Autodesk Fusion 360 part; units mm, degrees
(part 3 of 5)
  spline S141 degree 3 poles (-283.1906, 51.225) (-283.1957, 51.1131) (-283.2051, 50.9053) (-283.324, 50.7357) (-283.3788, 50.6575) knots 0 0 0 0 0.032809 0.060899 0.060899 0.060899 0.060899
  spline S142 degree 3 poles (-283.3788, 50.6575) (-283.4474, 50.5986) (-283.5878, 50.478) (-283.7726, 50.4631) (-283.8672, 50.4556) knots 0 0 0 0 0.026399 0.05408 0.05408 0.05408 0.05408
  spline S143 degree 3 poles (-283.8672, 50.4556) (-283.959, 50.4631) (-284.1388, 50.4779) (-284.2752, 50.5957) (-284.342, 50.6534) knots 0 0 0 0 0.026858 0.052633 0.052633 0.052633 0.052633
  spline S144 degree 3 poles (-284.342, 50.6534) (-284.3956, 50.7301) (-284.512, 50.8965) (-284.5212, 51.1002) (-284.5262, 51.21) knots 0 0 0 0 0.027523 0.05971 0.05971 0.05971 0.05971
  spline S145 degree 3 poles (-284.5262, 51.21) (-284.5261, 51.2191) (-284.5259, 51.2409) (-284.5252, 51.2627) (-284.5248, 51.2755) knots 0 0 0 0 0.002729 0.00655 0.00655 0.00655 0.00655
  line L105 (-284.5248, 51.2755) -> (-283.4443, 51.2755)
  spline S146 degree 3 poles (-283.4443, 51.2755) (-283.4514, 51.3482) (-283.4645, 51.4824) (-283.5433, 51.5913) (-283.5794, 51.6411) knots 0 0 0 0 0.021465 0.039604 0.039604 0.039604 0.039604
  spline S147 degree 3 poles (-283.5794, 51.6411) (-283.6226, 51.6781) (-283.7099, 51.7528) (-283.8244, 51.7629) (-283.8822, 51.768) knots 0 0 0 0 0.016633 0.033577 0.033577 0.033577 0.033577
  line L106 (-285.0691, 51.1786) -> (-285.0691, 51.9371)
  line L107 (-285.0691, 51.9371) -> (-284.8236, 51.9371)
  line L108 (-284.8236, 51.9371) -> (-284.8236, 50.4883)
  line L109 (-284.8236, 50.4883) -> (-285.0446, 50.4883)
  line L110 (-285.0446, 50.4883) -> (-285.0446, 50.7079)
  spline S148 degree 3 poles (-285.0446, 50.7079) (-285.0692, 50.6633) (-285.1111, 50.5874) (-285.1746, 50.5288) (-285.2008, 50.5047) knots 0 0 0 0 0.015158 0.025781 0.025781 0.025781 0.025781
  spline S149 degree 3 poles (-285.2008, 50.5047) (-285.2252, 50.4904) (-285.2739, 50.4618) (-285.3303, 50.4576) (-285.3584, 50.4556) knots 0 0 0 0 0.008374 0.016702 0.016702 0.016702 0.016702
  spline S150 degree 3 poles (-285.3584, 50.4556) (-285.4009, 50.4595) (-285.4906, 50.4677) (-285.5693, 50.5116) (-285.6107, 50.5347) knots 0 0 0 0 0.012672 0.02671 0.02671 0.02671 0.02671
  line L111 (-285.6107, 50.5347) -> (-285.5262, 50.7625)
  spline S151 degree 3 poles (-285.5262, 50.7625) (-285.4968, 50.747) (-285.4403, 50.7172) (-285.3766, 50.7119) (-285.3461, 50.7093) knots 0 0 0 0 0.009849 0.018951 0.018951 0.018951 0.018951
  spline S152 degree 3 poles (-285.3461, 50.7093) (-285.3199, 50.7113) (-285.2677, 50.7154) (-285.2235, 50.7436) (-285.2015, 50.7577) knots 0 0 0 0 0.007735 0.015463 0.015463 0.015463 0.015463
  spline S153 degree 3 poles (-285.2015, 50.7577) (-285.1815, 50.7759) (-285.1403, 50.8133) (-285.1203, 50.8653) (-285.1101, 50.8921) knots 0 0 0 0 0.007973 0.016455 0.016455 0.016455 0.016455
  spline S154 degree 3 poles (-285.1101, 50.8921) (-285.0981, 50.9376) (-285.0735, 51.0315) (-285.0706, 51.1285) (-285.0691, 51.1786) knots 0 0 0 0 0.01405 0.029024 0.029024 0.029024 0.029024
  line L112 (-278.1333, 51.124) -> (-278.1333, 51.9371)
  line L113 (-278.1333, 51.9371) -> (-277.8686, 51.9371)
  line L114 (-277.8686, 51.9371) -> (-277.8686, 49.9371)
  line L115 (-277.8686, 49.9371) -> (-278.623, 49.9371)
  spline S155 degree 3 poles (-278.623, 49.9371) (-278.6817, 49.9373) (-278.7835, 49.9376) (-278.8844, 49.9507) (-278.9272, 49.9562) knots 0 0 0 0 0.017571 0.030509 0.030509 0.030509 0.030509
  spline S156 degree 3 poles (-278.9272, 49.9562) (-278.9734, 49.9656) (-279.0608, 49.9833) (-279.1378, 50.0284) (-279.1742, 50.0497) knots 0 0 0 0 0.014001 0.026564 0.026564 0.026564 0.026564
  spline S157 degree 3 poles (-279.1742, 50.0497) (-279.2061, 50.0756) (-279.2722, 50.1294) (-279.3132, 50.2041) (-279.3345, 50.2427) knots 0 0 0 0 0.012214 0.025303 0.025303 0.025303 0.025303
  spline S158 degree 3 poles (-279.3345, 50.2427) (-279.3522, 50.2856) (-279.3883, 50.373) (-279.3929, 50.4675) (-279.3952, 50.5156) knots 0 0 0 0 0.013801 0.028138 0.028138 0.028138 0.028138
  spline S159 degree 3 poles (-279.3952, 50.5156) (-279.3889, 50.5968) (-279.3765, 50.7566) (-279.2802, 50.8845) (-279.2328, 50.9474) knots 0 0 0 0 0.023898 0.046996 0.046996 0.046996 0.046996
  spline S160 degree 3 poles (-279.2328, 50.9474) (-279.1593, 50.9986) (-278.9848, 51.1201) (-278.7703, 51.1226) (-278.6462, 51.124) knots 0 0 0 0 0.026356 0.062507 0.062507 0.062507 0.062507
  line L116 (-278.6462, 51.124) -> (-278.1333, 51.124)
  spline S161 degree 3 poles (-257.0244, 103.3904) (-257.0362, 103.3956) (-257.0628, 103.4073) (-257.092, 103.4078) (-257.1083, 103.4081) knots 0 0 0 0 0.003804 0.008651 0.008651 0.008651 0.008651
  spline S162 degree 3 poles (-257.1083, 103.4081) (-257.1242, 103.4076) (-257.1603, 103.4063) (-257.196, 103.4014) (-257.2161, 103.3986) knots 0 0 0 0 0.004747 0.010826 0.010826 0.010826 0.010826
  line L117 (-257.2161, 103.3986) -> (-257.2516, 103.6155)
  spline S163 degree 3 poles (-257.2516, 103.6155) (-257.219, 103.6219) (-257.1576, 103.6338) (-257.0952, 103.6362) (-257.0661, 103.6373) knots 0 0 0 0 0.009958 0.018706 0.018706 0.018706 0.018706
  spline S164 degree 3 poles (-257.0661, 103.6373) (-257.0259, 103.6366) (-256.954, 103.6352) (-256.8879, 103.6073) (-256.8587, 103.595) knots 0 0 0 0 0.011916 0.021334 0.021334 0.021334 0.021334
  spline S165 degree 3 poles (-256.8587, 103.595) (-256.8361, 103.5802) (-256.7925, 103.5516) (-256.7672, 103.5059) (-256.755, 103.4839) knots 0 0 0 0 0.007958 0.015408 0.015408 0.015408 0.015408
  spline S166 degree 3 poles (-256.755, 103.4839) (-256.7464, 103.4484) (-256.7233, 103.3534) (-256.7243, 103.2553) (-256.725, 103.194) knots 0 0 0 0 0.010927 0.02924 0.02924 0.02924 0.02924
  line L118 (-256.725, 103.194) -> (-256.725, 102.3604)
  line L119 (-256.725, 102.3604) -> (-256.5449, 102.3604)
  line L120 (-256.5449, 102.3604) -> (-256.5449, 102.1694)
  line L121 (-256.5449, 102.1694) -> (-256.725, 102.1694)
  line L122 (-256.725, 102.1694) -> (-256.725, 101.8106)
  line L123 (-256.725, 101.8106) -> (-256.9692, 101.6633)
  line L124 (-256.9692, 101.6633) -> (-256.9692, 102.1694)
  line L125 (-256.9692, 102.1694) -> (-257.2161, 102.1694)
  line L126 (-257.2161, 102.1694) -> (-257.2161, 102.3604)
  line L127 (-257.2161, 102.3604) -> (-256.9692, 102.3604)
  line L128 (-256.9692, 102.3604) -> (-256.9692, 103.2076)
  spline S167 degree 3 poles (-256.9692, 103.2076) (-256.9688, 103.2365) (-256.9683, 103.2821) (-256.9784, 103.3265) (-256.9822, 103.3427) knots 0 0 0 0 0.008635 0.013608 0.013608 0.013608 0.013608
  spline S168 degree 3 poles (-256.9822, 103.3427) (-256.9872, 103.3522) (-256.9975, 103.3715) (-257.0154, 103.384) (-257.0244, 103.3904) knots 0 0 0 0 0.003189 0.00646 0.00646 0.00646 0.00646
  spline S169 degree 3 poles (-252.8144, 103.5848) (-252.7657, 103.5945) (-252.6592, 103.6158) (-252.5506, 103.6174) (-252.4917, 103.6182) knots 0 0 0 0 0.014862 0.032497 0.032497 0.032497 0.032497
  line L129 (-252.4917, 103.6182) -> (-251.7291, 103.6182)
  line L130 (-251.7291, 103.6182) -> (-251.7291, 101.6182)
  line L131 (-251.7291, 101.6182) -> (-252.4794, 101.6182)
  spline S170 degree 3 poles (-252.4794, 101.6182) (-252.5489, 101.6195) (-252.6746, 101.6218) (-252.7938, 101.6613) (-252.8471, 101.6789) knots 0 0 0 0 0.020707 0.037453 0.037453 0.037453 0.037453
  spline S171 degree 3 poles (-252.8471, 101.6789) (-252.8907, 101.7018) (-252.9775, 101.7473) (-253.0353, 101.8265) (-253.064, 101.8658) knots 0 0 0 0 0.014555 0.028975 0.028975 0.028975 0.028975
  spline S172 degree 3 poles (-253.064, 101.8658) (-253.0869, 101.9079) (-253.1317, 101.9904) (-253.1389, 102.084) (-253.1425, 102.1298) knots 0 0 0 0 0.014187 0.027818 0.027818 0.027818 0.027818
  spline S173 degree 3 poles (-253.1425, 102.1298) (-253.1394, 102.1721) (-253.1334, 102.2575) (-253.0932, 102.3331) (-253.0729, 102.3713) knots 0 0 0 0 0.01257 0.025379 0.025379 0.025379 0.025379
  spline S174 degree 3 poles (-253.0729, 102.3713) (-253.0458, 102.4077) (-252.9891, 102.4838) (-252.9061, 102.53) (-252.8628, 102.5541) knots 0 0 0 0 0.013451 0.028132 0.028132 0.028132 0.028132
  spline S175 degree 3 poles (-252.8628, 102.5541) (-252.919, 102.574) (-253.0268, 102.6121) (-253.1046, 102.6956) (-253.1418, 102.7356) knots 0 0 0 0 0.017587 0.033722 0.033722 0.033722 0.033722
  spline S176 degree 3 poles (-253.1418, 102.7356) (-253.1702, 102.7808) (-253.2284, 102.8734) (-253.2356, 102.9826) (-253.2393, 103.0384) knots 0 0 0 0 0.015782 0.032266 0.032266 0.032266 0.032266
  spline S177 degree 3 poles (-253.2393, 103.0384) (-253.237, 103.0842) (-253.2323, 103.1747) (-253.1973, 103.2584) (-253.18, 103.2997) knots 0 0 0 0 0.013638 0.026971 0.026971 0.026971 0.026971
  spline S178 degree 3 poles (-253.18, 103.2997) (-253.1599, 103.3369) (-253.1218, 103.4076) (-253.0617, 103.4608) (-253.0333, 103.4859) knots 0 0 0 0 0.012583 0.02387 0.02387 0.02387 0.02387
  spline S179 degree 3 poles (-253.0333, 103.4859) (-253.0013, 103.5067) (-252.9333, 103.5507) (-252.8555, 103.573) (-252.8144, 103.5848) knots 0 0 0 0 0.011395 0.024144 0.024144 0.024144 0.024144
  spline S180 degree 3 poles (-269.284, 103.5337) (-269.2388, 103.4878) (-269.1427, 103.3903) (-269.1115, 103.2566) (-269.095, 103.1858) knots 0 0 0 0 0.01895 0.040278 0.040278 0.040278 0.040278
  line L132 (-269.095, 103.1858) -> (-269.3379, 103.1476)
  spline S181 degree 3 poles (-269.713, 103.4491) (-269.7635, 103.4479) (-269.8534, 103.4458) (-269.9303, 103.4002) (-269.9641, 103.3802) knots 0 0 0 0 0.014834 0.026419 0.026419 0.026419 0.026419
  spline S182 degree 3 poles (-269.9641, 103.3802) (-269.9879, 103.3569) (-270.0338, 103.3122) (-270.042, 103.2489) (-270.0459, 103.2185) knots 0 0 0 0 0.009682 0.0186 0.0186 0.0186 0.0186
  spline S183 degree 3 poles (-269.4572, 102.166) (-269.4912, 102.1574) (-269.5609, 102.1399) (-269.6326, 102.1378) (-269.6694, 102.1367) knots 0 0 0 0 0.010482 0.021472 0.021472 0.021472 0.021472
  spline S184 degree 3 poles (-269.6694, 102.1367) (-269.7232, 102.1382) (-269.8253, 102.1412) (-269.9227, 102.1715) (-269.9688, 102.1858) knots 0 0 0 0 0.01606 0.030471 0.030471 0.030471 0.030471
  spline S185 degree 3 poles (-268.4797, 103.3781) (-268.5106, 103.349) (-268.5781, 103.2853) (-268.6125, 103.1987) (-268.6312, 103.1517) knots 0 0 0 0 0.012573 0.027537 0.027537 0.027537 0.027537
  line L133 (-268.6312, 103.1517) -> (-268.8849, 103.183)
  line L134 (-252.4198, 62.5518) -> (-336.4198, 62.5518)
  line L135 (-336.4198, 62.5518) -> (-336.4198, 86.5518)
  line L136 (-336.4198, 86.5518) -> (-252.4198, 86.5518)
  line L137 (-252.4198, 86.5518) -> (-252.4198, 62.5518)
  line L138 (-334.4198, 84.5518) -> (-254.4198, 84.5518)
  line L139 (-254.4198, 84.5518) -> (-254.4198, 64.5518)
  line L140 (-254.4198, 64.5518) -> (-334.4198, 64.5518)
  line L141 (-334.4198, 64.5518) -> (-334.4198, 84.5518)
  line L142 (-254.4198, 64.5518) -> (-264.4198, 64.5518)
  line L143 (-264.4198, 64.5518) -> (-264.4198, 74.5518)
  line L144 (-264.4198, 74.5518) -> (-254.4198, 74.5518)
  line L145 (-254.4198, 74.5518) -> (-254.4198, 64.5518)
  line L146 (-264.4198, 74.5518) -> (-274.4198, 74.5518)
  line L147 (-274.4198, 74.5518) -> (-274.4198, 64.5518)
  line L148 (-274.4198, 64.5518) -> (-264.4198, 64.5518)
  line L149 (-264.4198, 64.5518) -> (-264.4198, 74.5518)
  line L150 (-274.4198, 74.5518) -> (-284.4198, 74.5518)
  line L151 (-284.4198, 74.5518) -> (-284.4198, 64.5518)
  line L152 (-284.4198, 64.5518) -> (-274.4198, 64.5518)
  line L153 (-274.4198, 64.5518) -> (-274.4198, 74.5518)
  line L154 (-284.4198, 74.5518) -> (-294.4198, 74.5518)
  line L155 (-294.4198, 74.5518) -> (-294.4198, 64.5518)
  line L156 (-294.4198, 64.5518) -> (-284.4198, 64.5518)
  line L157 (-284.4198, 64.5518) -> (-284.4198, 74.5518)
  line L158 (-294.4198, 74.5518) -> (-304.4198, 74.5518)
  line L159 (-304.4198, 74.5518) -> (-304.4198, 64.5518)
  line L160 (-304.4198, 64.5518) -> (-294.4198, 64.5518)
  line L161 (-294.4198, 64.5518) -> (-294.4198, 74.5518)
  line L162 (-304.4198, 74.5518) -> (-314.4198, 74.5518)
  line L163 (-314.4198, 74.5518) -> (-314.4198, 64.5518)
  line L164 (-314.4198, 64.5518) -> (-304.4198, 64.5518)
  line L165 (-304.4198, 64.5518) -> (-304.4198, 74.5518)
  line L166 (-314.4198, 74.5518) -> (-324.4198, 74.5518)
  line L167 (-324.4198, 64.5518) -> (-314.4198, 64.5518)
  line L168 (-314.4198, 64.5518) -> (-314.4198, 74.5518)
  line L169 (-324.4198, 74.5518) -> (-334.4198, 74.5518)
  line L170 (-334.4198, 74.5518) -> (-334.4198, 64.5518)
  line L171 (-334.4198, 64.5518) -> (-324.4198, 64.5518)
  line L172 (-254.4198, 64.5518) -> (-264.4198, 64.5518)
  line L173 (-264.4198, 64.5518) -> (-264.4198, 74.5518)
  line L174 (-264.4198, 74.5518) -> (-254.4198, 74.5518)
  line L175 (-254.4198, 74.5518) -> (-254.4198, 64.5518)
  line L176 (-254.4198, 64.5518) -> (-264.4198, 74.5518)
  line L177 (-264.4198, 74.5518) -> (-274.4198, 64.5518)
  line L178 (-274.4198, 64.5518) -> (-284.4198, 74.5518)
  line L179 (-284.4198, 74.5518) -> (-294.4198, 64.5518)
  line L180 (-294.4198, 64.5518) -> (-304.4198, 74.5518)
  line L181 (-304.4198, 74.5518) -> (-314.4198, 64.5518)
  line L182 (-314.4198, 64.5518) -> (-324.4198, 74.5518)
  line L183 (-324.4198, 74.5518) -> (-334.4198, 64.5518)
  line L184 (-262.0056, 73.5518) -> (-255.4198, 73.5518)
  line L185 (-255.4198, 73.5518) -> (-255.4198, 66.966)
  line L186 (-255.4198, 66.966) -> (-262.0056, 73.5518)
  line L187 (-256.834, 65.5518) -> (-263.4198, 72.1376)
  line L188 (-263.4198, 65.5518) -> (-263.4198, 72.1376)
  line L189 (-256.834, 65.5518) -> (-263.4198, 65.5518)
  line L190 (-272.0056, 65.5518) -> (-265.4198, 65.5518)
  line L191 (-265.4198, 65.5518) -> (-265.4198, 72.1376)
  line L192 (-265.4198, 72.1376) -> (-272.0056, 65.5518)
  line L193 (-273.4198, 73.5518) -> (-273.4198, 66.966)
  line L194 (-266.834, 73.5518) -> (-273.4198, 66.966)
  line L195 (-266.834, 73.5518) -> (-273.4198, 73.5518)
  line L196 (-275.4198, 73.5518) -> (-275.4198, 66.966)
  line L197 (-275.4198, 66.966) -> (-282.0056, 73.5518)
  line L198 (-275.4198, 73.5518) -> (-282.0056, 73.5518)
  line L199 (-283.4198, 72.1376) -> (-283.4198, 65.5518)
  line L200 (-283.4198, 65.5518) -> (-276.834, 65.5518)
  line L201 (-276.834, 65.5518) -> (-283.4198, 72.1376)
  line L202 (-292.0056, 65.5518) -> (-285.4198, 65.5518)
  line L203 (-285.4198, 65.5518) -> (-285.4198, 72.1376)
  line L204 (-285.4198, 72.1376) -> (-292.0056, 65.5518)
  line L205 (-293.4198, 73.5518) -> (-293.4198, 66.966)
  line L206 (-286.834, 73.5518) -> (-293.4198, 66.966)
  line L207 (-286.834, 73.5518) -> (-293.4198, 73.5518)
  line L208 (-295.4198, 73.5518) -> (-295.4198, 66.966)
  line L209 (-295.4198, 66.966) -> (-302.0056, 73.5518)
  line L210 (-295.4198, 73.5518) -> (-302.0056, 73.5518)
  line L211 (-303.4198, 65.5518) -> (-303.4198, 72.1376)
  line L212 (-304.4198, 64.5518) -> (-304.4198, 65.5518)
  line L213 (-303.4198, 65.5518) -> (-296.834, 65.5518)
  line L214 (-296.834, 65.5518) -> (-303.4198, 72.1376)
  line L215 (-305.4198, 65.5518) -> (-305.4198, 72.1376)
  line L216 (-305.4198, 72.1376) -> (-312.0056, 65.5518)
  line L217 (-312.0056, 65.5518) -> (-305.4198, 65.5518)
  line L218 (-306.834, 73.5518) -> (-313.4198, 73.5518)
  line L219 (-313.4198, 66.966) -> (-313.4198, 73.5518)
  line L220 (-306.834, 73.5518) -> (-313.4198, 66.966)
  line L221 (-315.4198, 73.5518) -> (-322.0056, 73.5518)
  line L222 (-315.4198, 66.966) -> (-322.0056, 73.5518)
  line L223 (-315.4198, 73.5518) -> (-315.4198, 66.966)
  line L224 (-316.834, 65.5518) -> (-323.4198, 72.1376)
  line L225 (-323.4198, 72.1376) -> (-323.4198, 65.5518)
  line L226 (-323.4198, 65.5518) -> (-316.834, 65.5518)
  line L227 (-325.4198, 72.1376) -> (-332.0056, 65.5518)
  line L228 (-325.4198, 72.1376) -> (-325.4198, 65.5518)
  line L229 (-325.4198, 65.5518) -> (-332.0056, 65.5518)
  line L230 (-333.4198, 73.5518) -> (-333.4198, 66.966)
  line L231 (-326.834, 73.5518) -> (-333.4198, 66.966)
  line L232 (-326.834, 73.5518) -> (-333.4198, 73.5518)
  line L233 (-326.834, 75.5518) -> (-333.4198, 75.5518)
  line L234 (-306.834, 75.5518) -> (-313.4198, 75.5518)
  line L235 (-315.4198, 75.5518) -> (-322.0056, 75.5518)
  line L236 (-295.4198, 75.5518) -> (-302.0056, 75.5518)
  line L237 (-286.834, 75.5518) -> (-293.4198, 75.5518)
  line L238 (-275.4198, 75.5518) -> (-282.0056, 75.5518)
  line L239 (-283.4198, 83.5518) -> (-276.834, 83.5518)
  line L240 (-325.4198, 83.5518) -> (-332.0056, 83.5518)
  line L241 (-292.0056, 83.5518) -> (-285.4198, 83.5518)
  line L242 (-303.4198, 83.5518) -> (-296.834, 83.5518)
  line L243 (-256.834, 83.5518) -> (-263.4198, 83.5518)
  line L244 (-325.4198, 76.966) -> (-332.0056, 83.5518)
  line L245 (-323.4198, 83.5518) -> (-316.834, 83.5518)
  line L246 (-266.834, 75.5518) -> (-273.4198, 75.5518)
  line L247 (-333.4198, 75.5518) -> (-333.4198, 82.1376)
  line L248 (-312.0056, 83.5518) -> (-305.4198, 83.5518)
  line L249 (-326.834, 75.5518) -> (-333.4198, 82.1376)
  line L250 (-305.4198, 76.966) -> (-312.0056, 83.5518)
  line L251 (-272.0056, 83.5518) -> (-265.4198, 83.5518)
  line L252 (-276.834, 83.5518) -> (-283.4198, 76.966)
  line L253 (-315.4198, 75.5518) -> (-315.4198, 82.1376)
  line L254 (-255.4198, 82.1376) -> (-262.0056, 75.5518)
  line L255 (-293.4198, 75.5518) -> (-293.4198, 82.1376)
  line L256 (-283.4198, 76.966) -> (-283.4198, 83.5518)
  line L257 (-285.4198, 76.966) -> (-292.0056, 83.5518)
  line L258 (-275.4198, 82.1376) -> (-282.0056, 75.5518)
  line L259 (-275.4198, 75.5518) -> (-275.4198, 82.1376)
  line L260 (-296.834, 83.5518) -> (-303.4198, 76.966)
  line L261 (-323.4198, 76.966) -> (-323.4198, 83.5518)
  line L262 (-285.4198, 83.5518) -> (-285.4198, 76.966)
  line L263 (-273.4198, 75.5518) -> (-273.4198, 82.1376)
  line L264 (-313.4198, 82.1376) -> (-313.4198, 75.5518)
  line L265 (-262.0056, 75.5518) -> (-255.4198, 75.5518)
  line L266 (-286.834, 75.5518) -> (-293.4198, 82.1376)
  line L267 (-255.4198, 75.5518) -> (-255.4198, 82.1376)
  line L268 (-305.4198, 83.5518) -> (-305.4198, 76.966)
  line L269 (-265.4198, 83.5518) -> (-265.4198, 76.966)
  line L270 (-265.4198, 76.966) -> (-272.0056, 83.5518)
  line L271 (-325.4198, 76.966) -> (-325.4198, 83.5518)
  line L272 (-316.834, 83.5518) -> (-323.4198, 76.966)
  line L273 (-266.834, 75.5518) -> (-273.4198, 82.1376)
  line L274 (-256.834, 83.5518) -> (-263.4198, 76.966)
  line L275 (-306.834, 75.5518) -> (-313.4198, 82.1376)
  line L276 (-295.4198, 75.5518) -> (-295.4198, 82.1376)
  line L277 (-303.4198, 83.5518) -> (-303.4198, 76.966)
  line L278 (-263.4198, 83.5518) -> (-263.4198, 76.966)
  line L279 (-295.4198, 82.1376) -> (-302.0056, 75.5518)
  line L280 (-315.4198, 82.1376) -> (-322.0056, 75.5518)
  line L281 (-265.6571, 101.6182) -> (-266.5439, 101.6182)
  spline S186 degree 3 poles (-267.5384, 51.7255) (-267.4544, 51.7234) (-267.2987, 51.7194) (-267.1513, 51.6694) (-267.0834, 51.6464) knots 0 0 0 0 0.025027 0.046416 0.046416 0.046416 0.046416
  spline S187 degree 3 poles (-269.7144, 103.651) (-269.6293, 103.6486) (-269.4757, 103.6442) (-269.3431, 103.5678) (-269.284, 103.5337) knots 0 0 0 0 0.025053 0.045234 0.045234 0.045234 0.045234
  spline S188 degree 3 poles (-269.3379, 103.1476) (-269.3468, 103.1926) (-269.3638, 103.2781) (-269.4235, 103.3414) (-269.4518, 103.3713) knots 0 0 0 0 0.013461 0.025563 0.025563 0.025563 0.025563
  spline S189 degree 3 poles (-269.4518, 103.3713) (-269.4881, 103.3939) (-269.5678, 103.4435) (-269.6619, 103.4471) (-269.713, 103.4491) knots 0 0 0 0 0.012631 0.027679 0.027679 0.027679 0.027679
  spline S190 degree 3 poles (-270.0459, 103.2185) (-270.0428, 103.1922) (-270.0364, 103.1388) (-269.9947, 103.1048) (-269.9736, 103.0875) knots 0 0 0 0 0.007652 0.015492 0.015492 0.015492 0.015492
  spline S191 degree 3 poles (-269.9736, 103.0875) (-269.9445, 103.0745) (-269.8638, 103.0382) (-269.7777, 103.0175) (-269.7226, 103.0043) knots 0 0 0 0 0.009553 0.026493 0.026493 0.026493 0.026493
  spline S192 degree 3 poles (-269.7226, 103.0043) (-269.6457, 102.9851) (-269.5185, 102.9532) (-269.3964, 102.9053) (-269.3481, 102.8863) knots 0 0 0 0 0.023736 0.039299 0.039299 0.039299 0.039299
  spline S193 degree 3 poles (-269.3481, 102.8863) (-269.3157, 102.8686) (-269.2528, 102.8342) (-269.2104, 102.7765) (-269.1898, 102.7485) knots 0 0 0 0 0.010927 0.021211 0.021211 0.021211 0.021211
  spline S194 degree 3 poles (-269.1898, 102.7485) (-269.1741, 102.7183) (-269.1424, 102.6573) (-269.1381, 102.5887) (-269.1359, 102.5541) knots 0 0 0 0 0.010103 0.020373 0.020373 0.020373 0.020373
  spline S195 degree 3 poles (-269.1359, 102.5541) (-269.1377, 102.5225) (-269.1413, 102.46) (-269.1674, 102.403) (-269.1803, 102.3747) knots 0 0 0 0 0.009394 0.018625 0.018625 0.018625 0.018625
  spline S196 degree 3 poles (-269.1803, 102.3747) (-269.1964, 102.3484) (-269.2287, 102.2956) (-269.2769, 102.257) (-269.301, 102.2376) knots 0 0 0 0 0.009191 0.018392 0.018392 0.018392 0.018392
  spline S197 degree 3 poles (-269.301, 102.2376) (-269.3232, 102.2237) (-269.372, 102.1929) (-269.4271, 102.1755) (-269.4572, 102.166) knots 0 0 0 0 0.007816 0.017247 0.017247 0.017247 0.017247
  spline S198 degree 3 poles (-269.9688, 102.1858) (-270.0081, 102.2024) (-270.0811, 102.2333) (-270.1345, 102.2918) (-270.1591, 102.3188) knots 0 0 0 0 0.012608 0.023462 0.023462 0.023462 0.023462
  spline S199 degree 3 poles (-270.1591, 102.3188) (-270.1783, 102.3508) (-270.2199, 102.4204) (-270.2354, 102.5001) (-270.2437, 102.5432) knots 0 0 0 0 0.011092 0.024145 0.024145 0.024145 0.024145
  line L282 (-270.2437, 102.5432) -> (-270.0036, 102.5759)
  spline S200 degree 3 poles (-270.0036, 102.5759) (-269.996, 102.5411) (-269.9813, 102.4735) (-269.9324, 102.4249) (-269.9088, 102.4013) knots 0 0 0 0 0.010457 0.02025 0.02025 0.02025 0.02025
  spline S201 degree 3 poles (-269.9088, 102.4013) (-269.878, 102.3831) (-269.81, 102.3427) (-269.7306, 102.34) (-269.6871, 102.3386) knots 0 0 0 0 0.01057 0.023371 0.023371 0.023371 0.023371
  spline S202 degree 3 poles (-269.6871, 102.3386) (-269.6377, 102.339) (-269.5526, 102.3396) (-269.4772, 102.3783) (-269.4456, 102.3945) knots 0 0 0 0 0.014562 0.025087 0.025087 0.025087 0.025087
  spline S203 degree 3 poles (-269.4456, 102.3945) (-269.4246, 102.4131) (-269.3847, 102.4484) (-269.377, 102.5008) (-269.3733, 102.5255) knots 0 0 0 0 0.00814 0.015395 0.015395 0.015395 0.015395
  spline S204 degree 3 poles (-269.3733, 102.5255) (-269.3746, 102.541) (-269.3772, 102.5723) (-269.3946, 102.5983) (-269.4033, 102.6114) knots 0 0 0 0 0.004598 0.009239 0.009239 0.009239 0.009239
  spline S205 degree 3 poles (-269.4033, 102.6114) (-269.4156, 102.6243) (-269.4423, 102.6526) (-269.4781, 102.6684) (-269.4975, 102.6769) knots 0 0 0 0 0.005284 0.01157 0.01157 0.01157 0.01157
  spline S206 degree 3 poles (-269.4975, 102.6769) (-269.5217, 102.6845) (-269.5935, 102.7071) (-269.6662, 102.7267) (-269.7144, 102.7397) knots 0 0 0 0 0.007605 0.022583 0.022583 0.022583 0.022583
  spline S207 degree 3 poles (-269.7144, 102.7397) (-269.7886, 102.7594) (-269.9115, 102.792) (-270.0307, 102.8361) (-270.078, 102.8536) knots 0 0 0 0 0.023005 0.038118 0.038118 0.038118 0.038118
  spline S208 degree 3 poles (-270.078, 102.8536) (-270.1102, 102.8697) (-270.1733, 102.9012) (-270.2179, 102.9558) (-270.2396, 102.9825) knots 0 0 0 0 0.010681 0.020888 0.020888 0.020888 0.020888
  spline S209 degree 3 poles (-270.2396, 102.9825) (-270.2567, 103.0134) (-270.2928, 103.0787) (-270.2964, 103.1533) (-270.2983, 103.1926) knots 0 0 0 0 0.010453 0.022074 0.022074 0.022074 0.022074
  spline S210 degree 3 poles (-270.2983, 103.1926) (-270.2951, 103.2332) (-270.2887, 103.3156) (-270.2476, 103.3874) (-270.2267, 103.4238) knots 0 0 0 0 0.012054 0.024479 0.024479 0.024479 0.024479
  spline S211 degree 3 poles (-270.2267, 103.4238) (-270.1994, 103.4582) (-270.1431, 103.5295) (-270.0619, 103.5704) (-270.02, 103.5916) knots 0 0 0 0 0.013001 0.026908 0.026908 0.026908 0.026908
  spline S212 degree 3 poles (-270.02, 103.5916) (-269.9725, 103.6089) (-269.8738, 103.6449) (-269.7688, 103.6489) (-269.7144, 103.651) knots 0 0 0 0 0.015065 0.0313 0.0313 0.0313 0.0313
  spline S213 degree 3 poles (-268.2492, 103.4491) (-268.292, 103.4465) (-268.3747, 103.4416) (-268.4455, 103.3988) (-268.4797, 103.3781) knots 0 0 0 0 0.012642 0.024448 0.024448 0.024448 0.024448
  spline S214 degree 3 poles (-268.8849, 103.183) (-268.8616, 103.2523) (-268.8165, 103.3862) (-268.7127, 103.4819) (-268.6626, 103.5282) knots 0 0 0 0 0.021523 0.041652 0.041652 0.041652 0.041652
  spline S215 degree 3 poles (-268.8931, 102.8911) (-268.893, 102.9002) (-268.8928, 102.922) (-268.8921, 102.9438) (-268.8917, 102.9566) knots 0 0 0 0 0.002729 0.00655 0.00655 0.00655 0.00655
  line L283 (-268.8917, 102.9566) -> (-267.8113, 102.9566)
  spline S216 degree 3 poles (-267.8113, 102.9566) (-267.8184, 103.0293) (-267.8314, 103.1635) (-267.9102, 103.2724) (-267.9463, 103.3222) knots 0 0 0 0 0.021465 0.039604 0.039604 0.039604 0.039604
  spline S217 degree 3 poles (-267.9463, 103.3222) (-267.9896, 103.3592) (-268.0769, 103.4339) (-268.1914, 103.444) (-268.2492, 103.4491) knots 0 0 0 0 0.016633 0.033577 0.033577 0.033577 0.033577
  spline S218 degree 3 poles (-266.8222, 103.2021) (-266.7876, 103.1487) (-266.7268, 103.0548) (-266.66, 102.9652) (-266.6312, 102.9266) knots 0 0 0 0 0.019089 0.033538 0.033538 0.033538 0.033538
  spline S219 degree 3 poles (-266.6312, 102.9266) (-266.6086, 102.8983) (-266.5688, 102.8486) (-266.5185, 102.8097) (-266.4968, 102.7929) knots 0 0 0 0 0.010792 0.019015 0.019015 0.019015 0.019015
  spline S220 degree 3 poles (-266.4968, 102.7929) (-266.4772, 102.7812) (-266.4392, 102.7584) (-266.3967, 102.7458) (-266.3761, 102.7397) knots 0 0 0 0 0.006806 0.01324 0.01324 0.01324 0.01324
  spline S221 degree 3 poles (-266.3761, 102.7397) (-266.3563, 102.7369) (-266.3075, 102.7301) (-266.2581, 102.7301) (-266.2287, 102.7301) knots 0 0 0 0 0.005978 0.01478 0.01478 0.01478 0.01478
  line L284 (-272.1892, 103.194) -> (-272.1892, 102.3604)
  line L285 (-272.1892, 102.3604) -> (-272.0091, 102.3604)
  line L286 (-272.0091, 102.3604) -> (-272.0091, 102.1694)
  line L287 (-272.0091, 102.1694) -> (-272.1892, 102.1694)
  line L288 (-272.1892, 102.1694) -> (-272.1892, 101.8106)
  line L289 (-272.1892, 101.8106) -> (-272.4334, 101.6633)
  line L290 (-272.4334, 101.6633) -> (-272.4334, 102.1694)
  line L291 (-272.4334, 102.1694) -> (-272.6803, 102.1694)
  line L292 (-272.6803, 102.1694) -> (-272.6803, 102.3604)
  line L293 (-272.6803, 102.3604) -> (-272.4334, 102.3604)
  line L294 (-272.4334, 102.3604) -> (-272.4334, 103.2076)
  spline S222 degree 3 poles (-272.4463, 103.3427) (-272.4514, 103.3522) (-272.4616, 103.3715) (-272.4795, 103.384) (-272.4886, 103.3904) knots 0 0 0 0 0.003189 0.00646 0.00646 0.00646 0.00646
  spline S223 degree 3 poles (-271.1851, 102.1367) (-271.2768, 102.1442) (-271.4567, 102.159) (-271.593, 102.2768) (-271.6598, 102.3345) knots 0 0 0 0 0.026858 0.052633 0.052633 0.052633 0.052633
  spline S224 degree 3 poles (-271.6598, 102.3345) (-271.7135, 102.4112) (-271.8298, 102.5776) (-271.839, 102.7813) (-271.844, 102.8911) knots 0 0 0 0 0.027523 0.05971 0.05971 0.05971 0.05971
  spline S225 degree 3 poles (-271.844, 102.8911) (-271.8439, 102.9002) (-271.8437, 102.922) (-271.843, 102.9438) (-271.8426, 102.9566) knots 0 0 0 0 0.002729 0.00655 0.00655 0.00655 0.00655
  line L295 (-271.8426, 102.9566) -> (-270.7621, 102.9566)
  spline S226 degree 3 poles (-267.0834, 51.6464) (-267.0258, 51.6171) (-266.912, 51.5591) (-266.834, 51.4582) (-266.7955, 51.4083) knots 0 0 0 0 0.019136 0.037772 0.037772 0.037772 0.037772
  spline S227 degree 3 poles (-272.6639, 51.4786) (-272.6028, 51.5502) (-272.4816, 51.6924) (-272.2962, 51.7136) (-272.2041, 51.7242) knots 0 0 0 0 0.027153 0.053891 0.053891 0.053891 0.053891
  spline S228 degree 3 poles (-272.2041, 51.7242) (-272.1624, 51.7222) (-272.08, 51.7184) (-272.0028, 51.6894) (-271.9647, 51.6751) knots 0 0 0 0 0.012458 0.024577 0.024577 0.024577 0.024577
  spline S229 degree 3 poles (-271.9647, 51.6751) (-271.9308, 51.6587) (-271.8677, 51.6281) (-271.8212, 51.5758) (-271.7996, 51.5516) knots 0 0 0 0 0.01116 0.020794 0.020794 0.020794 0.020794
  spline S230 degree 3 poles (-271.7996, 51.5516) (-271.7829, 51.5246) (-271.7477, 51.4681) (-271.7321, 51.4034) (-271.7239, 51.3695) knots 0 0 0 0 0.009458 0.019838 0.019838 0.019838 0.019838
  spline S231 degree 3 poles (-271.7239, 51.3695) (-271.7196, 51.3384) (-271.709, 51.2624) (-271.7089, 51.1856) (-271.7089, 51.1403) knots 0 0 0 0 0.009413 0.022992 0.022992 0.022992 0.022992
  line L296 (-271.7089, 51.1403) -> (-271.7089, 50.2426)
  line L297 (-271.7089, 50.2426) -> (-271.9545, 50.2426)
  line L298 (-271.9545, 50.2426) -> (-271.9545, 51.0461)
  spline S232 degree 3 poles (-271.9545, 51.0461) (-271.9542, 51.0999) (-271.9538, 51.1867) (-271.9652, 51.2726) (-271.9695, 51.3053) knots 0 0 0 0 0.016103 0.02599 0.02599 0.02599 0.02599
  spline S233 degree 3 poles (-271.9695, 51.3053) (-271.9791, 51.3357) (-271.9981, 51.3954) (-272.0448, 51.437) (-272.0677, 51.4575) knots 0 0 0 0 0.009371 0.018407 0.018407 0.018407 0.018407
  spline S234 degree 3 poles (-272.0677, 51.4575) (-272.095, 51.4736) (-272.1521, 51.5073) (-272.2185, 51.5109) (-272.2533, 51.5127) knots 0 0 0 0 0.009358 0.019615 0.019615 0.019615 0.019615
  spline S235 degree 3 poles (-272.2533, 51.5127) (-272.2896, 51.5103) (-272.3625, 51.5055) (-272.4278, 51.4726) (-272.4606, 51.4561) knots 0 0 0 0 0.010803 0.021692 0.021692 0.021692 0.021692
  spline S236 degree 3 poles (-273.4129, 51.2208) (-273.4218, 51.2658) (-273.4388, 51.3513) (-273.4985, 51.4146) (-273.5268, 51.4445) knots 0 0 0 0 0.013461 0.025563 0.025563 0.025563 0.025563
  spline S237 degree 3 poles (-273.5268, 51.4445) (-273.5631, 51.4671) (-273.6428, 51.5167) (-273.7369, 51.5203) (-273.788, 51.5223) knots 0 0 0 0 0.012631 0.027679 0.027679 0.027679 0.027679
  spline S238 degree 3 poles (-273.788, 51.5223) (-273.8385, 51.5211) (-273.9284, 51.519) (-274.0053, 51.4734) (-274.0391, 51.4534) knots 0 0 0 0 0.014834 0.026419 0.026419 0.026419 0.026419
  spline S239 degree 3 poles (-274.0391, 51.4534) (-274.0629, 51.4301) (-274.1088, 51.3854) (-274.117, 51.3221) (-274.1209, 51.2917) knots 0 0 0 0 0.009682 0.0186 0.0186 0.0186 0.0186
  spline S240 degree 3 poles (-274.1209, 51.2917) (-274.1178, 51.2653) (-274.1114, 51.212) (-274.0697, 51.1779) (-274.0486, 51.1607) knots 0 0 0 0 0.007652 0.015492 0.015492 0.015492 0.015492
  spline S241 degree 3 poles (-274.0486, 51.1607) (-274.0195, 51.1477) (-273.9388, 51.1114) (-273.8527, 51.0907) (-273.7976, 51.0775) knots 0 0 0 0 0.009553 0.026493 0.026493 0.026493 0.026493
  spline S242 degree 3 poles (-273.7976, 51.0775) (-273.7207, 51.0583) (-273.5935, 51.0264) (-273.4714, 50.9785) (-273.4231, 50.9595) knots 0 0 0 0 0.023737 0.039299 0.039299 0.039299 0.039299
  spline S243 degree 3 poles (-273.4231, 50.9595) (-273.3907, 50.9418) (-273.3278, 50.9074) (-273.2854, 50.8497) (-273.2648, 50.8217) knots 0 0 0 0 0.010927 0.021211 0.021211 0.021211 0.021211
  spline S244 degree 3 poles (-273.2648, 50.8217) (-273.2491, 50.7915) (-273.2174, 50.7305) (-273.2131, 50.6619) (-273.211, 50.6273) knots 0 0 0 0 0.010103 0.020373 0.020373 0.020373 0.020373
  spline S245 degree 3 poles (-273.211, 50.6273) (-273.2127, 50.5957) (-273.2163, 50.5331) (-273.2424, 50.4762) (-273.2553, 50.4479) knots 0 0 0 0 0.009394 0.018625 0.018625 0.018625 0.018625
  spline S246 degree 3 poles (-273.2553, 50.4479) (-273.2714, 50.4216) (-273.3037, 50.3688) (-273.3519, 50.3301) (-273.376, 50.3108) knots 0 0 0 0 0.009191 0.018392 0.018392 0.018392 0.018392
  spline S247 degree 3 poles (-273.376, 50.3108) (-273.3982, 50.2969) (-273.447, 50.2661) (-273.5021, 50.2487) (-273.5322, 50.2392) knots 0 0 0 0 0.007816 0.017247 0.017247 0.017247 0.017247
  spline S248 degree 3 poles (-273.5322, 50.2392) (-273.5662, 50.2306) (-273.6359, 50.2131) (-273.7076, 50.2109) (-273.7444, 50.2098) knots 0 0 0 0 0.010482 0.021472 0.021472 0.021472 0.021472
  spline S249 degree 3 poles (-273.7444, 50.2098) (-273.7982, 50.2114) (-273.9003, 50.2144) (-273.9977, 50.2446) (-274.0438, 50.259) knots 0 0 0 0 0.01606 0.030471 0.030471 0.030471 0.030471
  spline S250 degree 3 poles (-274.0438, 50.259) (-274.0831, 50.2756) (-274.1561, 50.3065) (-274.2095, 50.3649) (-274.2342, 50.392) knots 0 0 0 0 0.012607 0.023462 0.023462 0.023462 0.023462
  spline S251 degree 3 poles (-274.2342, 50.392) (-274.2533, 50.4239) (-274.2949, 50.4935) (-274.3104, 50.5733) (-274.3187, 50.6164) knots 0 0 0 0 0.011092 0.024145 0.024145 0.024145 0.024145
  line L299 (-274.3187, 50.6164) -> (-274.0786, 50.6491)
  spline S252 degree 3 poles (-274.0786, 50.6491) (-274.071, 50.6143) (-274.0563, 50.5467) (-274.0075, 50.498) (-273.9838, 50.4745) knots 0 0 0 0 0.010457 0.02025 0.02025 0.02025 0.02025
  spline S253 degree 3 poles (-269.1796, 51.6887) (-269.1469, 51.6951) (-269.0856, 51.707) (-269.0232, 51.7094) (-268.994, 51.7105) knots 0 0 0 0 0.009958 0.018706 0.018706 0.018706 0.018706
  spline S254 degree 3 poles (-268.994, 51.7105) (-268.9539, 51.7098) (-268.882, 51.7084) (-268.8159, 51.6805) (-268.7867, 51.6682) knots 0 0 0 0 0.011916 0.021334 0.021334 0.021334 0.021334
  spline S255 degree 3 poles (-268.7867, 51.6682) (-268.7641, 51.6534) (-268.7204, 51.6248) (-268.6952, 51.5791) (-268.683, 51.557) knots 0 0 0 0 0.007958 0.015408 0.015408 0.015408 0.015408
  spline S256 degree 3 poles (-268.683, 51.557) (-268.6744, 51.5215) (-268.6513, 51.4265) (-268.6523, 51.3285) (-268.653, 51.2671) knots 0 0 0 0 0.010927 0.02924 0.02924 0.02924 0.02924
  line L300 (-268.653, 51.2671) -> (-268.653, 50.4336)
  line L301 (-268.653, 50.4336) -> (-268.4729, 50.4336)
  line L302 (-268.4729, 50.4336) -> (-268.4729, 50.2426)
  line L303 (-268.4729, 50.2426) -> (-268.653, 50.2426)
  line L304 (-268.653, 50.2426) -> (-268.653, 49.8838)
  line L305 (-268.653, 49.8838) -> (-268.8972, 49.7364)
  line L306 (-268.8972, 49.7364) -> (-268.8972, 50.2426)
  line L307 (-268.8972, 50.2426) -> (-269.1441, 50.2426)
  line L308 (-269.1441, 50.2426) -> (-269.1441, 50.4336)
  spline S257 degree 3 poles (-268.6626, 103.5282) (-268.6025, 103.564) (-268.475, 103.6399) (-268.3264, 103.6472) (-268.2478, 103.651) knots 0 0 0 0 0.020652 0.043844 0.043844 0.043844 0.043844
  spline S258 degree 3 poles (-268.2478, 103.651) (-268.1489, 103.6444) (-267.9598, 103.6319) (-267.8135, 103.5123) (-267.7437, 103.4552) knots 0 0 0 0 0.028913 0.055291 0.055291 0.055291 0.055291
  spline S259 degree 3 poles (-267.7437, 103.4552) (-267.6895, 103.3795) (-267.5723, 103.2161) (-267.5627, 103.0144) (-267.5575, 102.9061) knots 0 0 0 0 0.027351 0.059089 0.059089 0.059089 0.059089
  spline S260 degree 3 poles (-267.5575, 102.9061) (-267.5626, 102.7942) (-267.5721, 102.5864) (-267.6909, 102.4168) (-267.7458, 102.3386) knots 0 0 0 0 0.032809 0.060899 0.060899 0.060899 0.060899
  spline S261 degree 3 poles (-267.7458, 102.3386) (-267.8143, 102.2797) (-267.9548, 102.1591) (-268.1396, 102.1442) (-268.2342, 102.1367) knots 0 0 0 0 0.026399 0.05408 0.05408 0.05408 0.05408
  spline S262 degree 3 poles (-268.2342, 102.1367) (-268.3259, 102.1442) (-268.5058, 102.159) (-268.6422, 102.2768) (-268.7089, 102.3345) knots 0 0 0 0 0.026858 0.052633 0.052633 0.052633 0.052633
  spline S263 degree 3 poles (-268.7089, 102.3345) (-268.7626, 102.4112) (-268.8789, 102.5776) (-268.8881, 102.7813) (-268.8931, 102.8911) knots 0 0 0 0 0.027523 0.05971 0.05971 0.05971 0.05971
  point P0 (-304.4198, 83.5518)
  dimension "d119" = 84
  dimension "d120" = 24
  dimension "d121" = 2
  dimension "d122" = 10
  dimension "d123" = 10
  dimension "d124" = 10
  dimension "d125" = 10
  dimension "d126" = 10
  dimension "d127" = 10
  dimension "d128" = 10
  dimension "d129" = 10
  dimension "d130" = 10
  dimension "d131" = 10
  dimension "d132" = 10
  dimension "d133" = 10
  dimension "d134" = 10
  dimension "d135" = 1
  dimension "d136" = -1
  dimension "d137" = -1
  dimension "d138" = -1
  dimension "d139" = 1
  dimension "d140" = -1
  dimension "d141" = -1
  dimension "d142" = -1
  dimension "d143" = 1
  dimension "d145" = 1
  dimension "d146" = -1
  dimension "d147" = -1
  dimension "d148" = 1
  dimension "d151" = -1
  constraint horizontal L134
  constraint vertical L135
  constraint horizontal L136
  constraint vertical L137
  constraint coincident L27.end A35.end
  constraint horizontal L142
  constraint vertical L143
  constraint horizontal L144
  constraint vertical L145
  constraint horizontal L146
  constraint vertical L147
  constraint horizontal L148
  constraint vertical L149
  constraint horizontal L150
  constraint vertical L151
  constraint horizontal L152
  constraint vertical L153
  constraint horizontal L154
  constraint vertical L155
  constraint horizontal L156
  constraint vertical L157
  constraint horizontal L158
  constraint vertical L159
  constraint horizontal L160
  constraint vertical L161
  constraint horizontal L162
  constraint vertical L163
  constraint horizontal L164
  constraint vertical L165
  constraint horizontal L166
  constraint horizontal L167
  constraint vertical L168
  constraint horizontal L169
  constraint vertical L170
  constraint horizontal L171
  constraint horizontal L172
  constraint vertical L173
  constraint horizontal L174
  constraint vertical L175
  constraint perpendicular L176 L177
  constraint perpendicular L160 L212
  constraint perpendicular L211 L213
  constraint symmetric L169 L184.start L254.end
  constraint symmetric L169 L184.end L265.end
  constraint symmetric L169 L185.end L254.start
  constraint symmetric L169 L187.start L243.start
  constraint symmetric L169 L187.end L274.end
  constraint symmetric L169 L188.start L243.end
  constraint symmetric L169 L190.start L251.start
  constraint symmetric L169 L190.end L251.end
  constraint symmetric L169 L191.end L269.end
  constraint symmetric L169 L193.start L246.end
  constraint symmetric L169 L193.end L263.end
  constraint symmetric L169 L194.start L246.start
  constraint symmetric L169 L196.start L238.start
  constraint symmetric L169 L196.end L258.start
  constraint symmetric L169 L197.end L238.end
  constraint symmetric L169 L199.start L252.end
  constraint symmetric L169 L199.end L239.start
  constraint symmetric L169 L200.end L239.end
  constraint symmetric L169 L202.start L241.start
  constraint symmetric L169 L202.end L241.end
  constraint symmetric L169 L203.end L257.start
  constraint symmetric L169 L205.start L237.end
  constraint symmetric L169 L205.end L255.end
  constraint symmetric L169 L206.start L237.start
  constraint symmetric L169 L208.start L236.start
  constraint symmetric L169 L208.end L276.end
  constraint symmetric L169 L209.end L236.end
  constraint symmetric L169 L211.end L260.end
  constraint symmetric L169 L212.end P0
  constraint symmetric L169 L213.end L242.end
  constraint symmetric L169 L211.start L242.start
  constraint symmetric L169 L215.start L248.end
  constraint symmetric L169 L215.end L250.start
  constraint symmetric L169 L216.end L248.start
  constraint symmetric L169 L218.start L234.start
  constraint symmetric L169 L218.end L234.end
  constraint symmetric L169 L219.start L264.start
  constraint symmetric L169 L221.start L235.start
  constraint symmetric L169 L221.end L235.end
  constraint symmetric L169 L222.start L253.end
  constraint symmetric L169 L224.start L245.end
  constraint symmetric L169 L224.end L261.start
  constraint symmetric L169 L225.end L245.start
  constraint symmetric L169 L227.start L244.start
  constraint symmetric L169 L227.end L240.end
  constraint symmetric L169 L228.end L240.start
  constraint symmetric L169 L230.start L233.end
  constraint symmetric L169 L230.end L247.end
  constraint symmetric L169 L231.start L233.start
  measures "d119" distance of L27.end L134.end
  measures "d120" distance of L27.end A56.start
  measures "d122" distance of L139.end L142.end
  measures "d123" distance of L143.end L146.end
  measures "d124" distance of L143.end L142.end
  measures "d125" distance of L146.end L150.end
  measures "d126" distance of L146.end L147.end
  measures "d127" distance of L150.end L154.end
  measures "d128" distance of L150.end L151.end
  measures "d129" distance of L154.end L158.end
  measures "d130" distance of L154.end L155.end
  measures "d131" distance of L158.end L162.end
  measures "d132" distance of L158.end L159.end
  measures "d133" distance of L162.end L166.end
  measures "d134" distance of L162.end L163.end
  measures "d145" distance of L159.end L212.end
extrude "Extrude3" cut sketch "Sketch3" against normal blind 2 contours L184 L185 L186 | L187 L188 L189 | L190 L191 L192 | L193 L194 L195 | L196 L197 L198 | L199 L200 L201 | L202 L203 L204 | L205 L206 L207 | L208 L209 L210 | L211 L213 L214 | L215 L216 L217 | L218 L219 L220 | L221 L222 L223 | L224 L225 L226 | L227 L228 L229 | L230 L231 L232 | L233 L247 L249 | L234 L264 L275 | L235 L253 L280 | L236 L276 L279 | L237 L255 L266 | L238 L258 L259 | L239 L252 L256 | L240 L244 L271 | L241 L257 L262 | L242 L260 L277 | L243 L274 L278 | L245 L261 L272 | L246 L263 L273 | L248 L250 L268 | L251 L269 L270 | L254 L265 L267